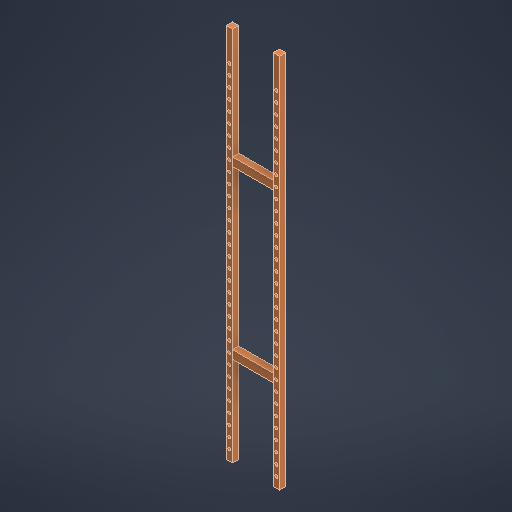
# Autodesk Inventor part: Probe_H_Frame
Saved by Autodesk Inventor 2027.1 (Build 311270010, 270A)
## iProperties
Created: 2026-09-21
Part Number: Probe_H_Frame
Material: Generic
Document SubType Name: Modeling
Designer: 박정현
Density: 1 g/cm^3
Appearance: Copper - grade unspecified
Author: 박정현
Comments: Reference-only H frame. Source: SO01373.10-Probe-R01.pdf, X2-X2. ASSUMED/EST parameters are not manufacturing dimensions. Four separate solids. M3 threads are nominal cylinders; no thread helix or unspecified fastening details.
Autodesk Inventor part; units mm, degrees
ref_plane "YZ Plane" through (0, 0, 0) normal (1, 0, 0) x (0, 1, 0)
ref_plane "XZ Plane" through (0, 0, 0) normal (0, 1, 0) x (-1, 0, 0)
ref_plane "XY Plane" through (0, 0, 0) normal (0, 0, 1) x (1, 0, 0)
sketch "Left_Rod_Profile" plane through (0, 0, 0) normal (0, 0, 1) x (1, 0, 0)
  line L0 (0, 0) -> (6, 0)
  line L1 (6, 0) -> (6, 360)
  line L2 (6, 360) -> (0, 360)
  line L3 (0, 360) -> (0, 0)
  dimension "d0" = 6
  dimension "d1" = 360
  constraints: 8 end point, 2 parallel, 1 coincident, 1 horizontal, 1 perpendicular
  measures "d0" distance of L1.end L2.end
  measures "d1" distance of L2.end L0.start
extrude "Left_Rod" add sketch "Left_Rod_Profile" along normal blind 6
sketch "Right_Rod_Profile" plane through (0, 0, 0) normal (0, 0, 1) x (1, 0, 0)
  line L0 (45, 0) -> (51, 0)
  line L1 (51, 0) -> (51, 360)
  line L2 (51, 360) -> (45, 360)
  line L3 (45, 360) -> (45, 0)
  point P0 (0, 0)
  dimension "d4" = 45
  dimension "d5" = 6
  dimension "d6" = 360
  constraints: 8 end point, 2 parallel, 1 horizontal, 1 horizontal alignment, 1 perpendicular
  measures "d4" distance of point (0, 0) L0.start
  measures "d5" distance of L1.end L2.end
  measures "d6" distance of L2.end L0.start
extrude "Right_Rod" add sketch "Right_Rod_Profile" along normal blind 6 separate body
sketch "Upper_Crossbar_ESTIMATED_Profile" plane through (0, 0, 0) normal (0, 0, 1) x (1, 0, 0)
  line L0 (6, 246) -> (45, 246)
  line L1 (45, 246) -> (45, 254)
  line L2 (45, 254) -> (6, 254)
  line L3 (6, 254) -> (6, 246)
  point P0 (0, 0)
  dimension "d9" = 6
  dimension "d10" = 246
  dimension "d11" = 39
  dimension "d12" = 8
  constraints: 8 end point, 2 parallel, 1 horizontal, 1 perpendicular
  measures "d9" horizontal distance of point (0, 0) L0.start
  measures "d10" vertical distance of point (0, 0) L0.start
  measures "d11" distance of L1.end L2.end
  measures "d12" distance of L2.end L0.start
extrude "Upper_Crossbar_ESTIMATED" add sketch "Upper_Crossbar_ESTIMATED_Profile" along normal blind 6 separate body
sketch "Lower_Crossbar_ESTIMATED_Profile" plane through (0, 0, 0) normal (0, 0, 1) x (1, 0, 0)
  line L0 (6, 86) -> (45, 86)
  line L1 (45, 86) -> (45, 94)
  line L2 (45, 94) -> (6, 94)
  line L3 (6, 94) -> (6, 86)
  point P0 (0, 0)
  dimension "d15" = 6
  dimension "d16" = 86
  dimension "d17" = 39
  dimension "d18" = 8
  constraints: 8 end point, 2 parallel, 1 horizontal, 1 perpendicular
  measures "d15" horizontal distance of point (0, 0) L0.start
  measures "d16" vertical distance of point (0, 0) L0.start
  measures "d17" distance of L1.end L2.end
  measures "d18" distance of L2.end L0.start
extrude "Lower_Crossbar_ESTIMATED" add sketch "Lower_Crossbar_ESTIMATED_Profile" along normal blind 6 separate body
sketch "M3_Nominal_Seed_Locations" plane through (0, 0, 0) normal (0, 0, 1) x (1, 0, 0)
  circle A0 centre (3, 330) radius 1.5
  circle A1 centre (48, 330) radius 1.5
  point P0 (0, 0)
  dimension "d21" = 3
  dimension "d22" = 330
  dimension "d23" = 3
  dimension "d24" = 48
  dimension "d25" = 330
  dimension "d26" = 3
  constraints: 2 centre point
  measures "d21" horizontal distance of point (0, 0) A0.centre
  measures "d22" vertical distance of point (0, 0) A0.centre
  measures "d23" diameter of A0
  measures "d24" horizontal distance of point (0, 0) A1.centre
  measures "d25" vertical distance of point (0, 0) A1.centre
  measures "d26" diameter of A1
extrude "M3_Simplified_Through_Seed" cut sketch "M3_Nominal_Seed_Locations" along normal through all bodies 1 2
pattern_linear "M3_33x_Per_Rod_10mm_Pitch" count 33 spacing 10 along (0, -1, 0) of "M3_Simplified_Through_Seed" bodies 1 2
equation "\"d0\" = RodWidth"
equation "\"d1\" = RodLength"
equation "\"d2\" = ASSUMED_RodDepth"
equation "\"d4\" = RodWidth + ClearGap"
equation "\"d5\" = RodWidth"
equation "\"d6\" = RodLength"
equation "\"d7\" = ASSUMED_RodDepth"
equation "\"d9\" = RodWidth"
equation "\"d10\" = -EST_UpperCrossbarFromTop + RodLength - 0.5 * EST_CrossbarHeight"
equation "\"d11\" = ClearGap"
equation "\"d12\" = EST_CrossbarHeight"
equation "\"d13\" = ASSUMED_CrossbarDepth"
equation "\"d15\" = RodWidth"
equation "\"d16\" = -EST_LowerCrossbarFromTop + RodLength - 0.5 * EST_CrossbarHeight"
equation "\"d17\" = ClearGap"
equation "\"d18\" = EST_CrossbarHeight"
equation "\"d19\" = ASSUMED_CrossbarDepth"
equation "\"d21\" = 0.5 * RodWidth"
equation "\"d22\" = RodLength - FirstHoleFromTop"
equation "\"d23\" = HoleNominalDiameter"
equation "\"d24\" = ClearGap + 1.5 * RodWidth"
equation "\"d25\" = RodLength - FirstHoleFromTop"
equation "\"d26\" = HoleNominalDiameter"
equation "\"RodLength\" = 360"
equation "\"RodWidth\" = 6"
equation "\"ClearGap\" = 39"
equation "\"ASSUMED_RodDepth\" = 6"
equation "\"ASSUMED_CrossbarDepth\" = 6"
equation "\"EST_CrossbarHeight\" = 8"
equation "\"FirstHoleFromTop\" = 30"
equation "\"HoleNominalDiameter\" = 3"
equation "\"OverallWidth\" = 2 * RodWidth + ClearGap"
equation "\"RodCentreSpacing\" = RodWidth + ClearGap"
equation "\"EST_UpperCrossbarFromTop\" = 110"
equation "\"EST_LowerCrossbarFromTop\" = 270"
body "Solid1"
body "Solid2"
body "Solid3"
body "Solid4"
